Autodesk Fusion 360 part; units mm, degrees
note: some values were not read from the file. Set by a fixed rule: which sketch regions a step uses.
(part 2 of 2)
sketch "Sketch6" plane through (0, 2, 0) normal (0, 1, 0) x (-1, 0, 0) in component "Case"
  arc A0 (-13.01, 94.472) -> (-15.51, 96.972) centre (-15.51, 94.472) ccw
  line L0 (-13.01, 94.472) -> (-13.01, 43.354)
  arc A1 (-13.01, 43.354) -> (-11.51, 41.854) centre (-11.51, 43.354) ccw
  line L1 (-11.51, 41.854) -> (2.524, 41.854)
  arc A2 (5.024, 39.354) -> (2.524, 41.854) centre (2.524, 39.354) ccw
  line L2 (5.024, 39.354) -> (5.024, -2.524)
  arc A3 (2.524, -5.024) -> (5.024, -2.524) centre (2.524, -2.524) ccw
  line L3 (2.524, -5.024) -> (-93.964, -5.024)
  arc A4 (-96.464, -2.524) -> (-93.964, -5.024) centre (-93.964, -2.524) ccw
  line L4 (-96.464, -2.524) -> (-96.464, 94.472)
  arc A5 (-93.964, 96.972) -> (-96.464, 94.472) centre (-93.964, 94.472) ccw
  line L5 (-93.964, 96.972) -> (-15.51, 96.972)
  line L6 (-10.51, 44.354) -> (-10.51, 94.472)
  arc A6 (-10.51, 94.472) -> (-15.51, 99.472) centre (-15.51, 94.472) ccw
  line L7 (-15.51, 99.472) -> (-93.964, 99.472)
  arc A7 (-93.964, 99.472) -> (-98.964, 94.472) centre (-93.964, 94.472) ccw
  line L8 (-98.964, 94.472) -> (-98.964, -2.524)
  arc A8 (-98.964, -2.524) -> (-93.964, -7.524) centre (-93.964, -2.524) ccw
  line L9 (-93.964, -7.524) -> (2.524, -7.524)
  arc A9 (2.524, -7.524) -> (7.524, -2.524) centre (2.524, -2.524) ccw
  line L10 (7.524, -2.524) -> (7.524, 39.354)
  arc A10 (7.524, 39.354) -> (2.524, 44.354) centre (2.524, 39.354) ccw
  line L11 (2.524, 44.354) -> (-10.51, 44.354)
  line L12 (-12.247, -4.524) -> (-12.247, -2.174)
  line L13 (-3.247, -2.174) -> (-3.247, -4.524)
  line L14 (-3.247, -4.524) -> (2.524, -4.524)
  arc A11 (2.524, -4.524) -> (4.524, -2.524) centre (2.524, -2.524) ccw
  line L15 (4.524, -2.524) -> (4.524, 39.354)
  arc A12 (4.524, 39.354) -> (2.524, 41.354) centre (2.524, 39.354) ccw
  line L16 (2.524, 41.354) -> (-11.51, 41.354)
  arc A13 (-13.51, 43.354) -> (-11.51, 41.354) centre (-11.51, 43.354) ccw
  line L17 (-13.51, 43.354) -> (-13.51, 94.472)
  arc A14 (-13.51, 94.472) -> (-15.51, 96.472) centre (-15.51, 94.472) ccw
  line L18 (-15.51, 96.472) -> (-93.964, 96.472)
  arc A15 (-93.964, 96.472) -> (-95.964, 94.472) centre (-93.964, 94.472) ccw
  line L19 (-95.964, 94.472) -> (-95.964, -2.524)
  arc A16 (-95.964, -2.524) -> (-93.964, -4.524) centre (-93.964, -2.524) ccw
  line L20 (-93.964, -4.524) -> (-12.247, -4.524)
  line L21 (-90.666, 67.049) -> (-90.666, 82.049)
  line L22 (-90.666, 82.049) -> (-76.466, 82.049)
  line L23 (-76.466, 82.049) -> (-76.466, 67.049)
  line L24 (-76.466, 67.049) -> (-90.666, 67.049)
  circle A17 centre (-20.066, 74.613) radius 1.5875
  circle A18 centre (-89.408, 55.499) radius 1.5875
  line L25 (-52.966, 38.874) -> (-52.966, 53.074)
  line L26 (-52.966, 53.074) -> (-37.966, 53.074)
  line L27 (-37.966, 53.074) -> (-37.966, 38.874)
  line L28 (-37.966, 38.874) -> (-52.966, 38.874)
  line L29 (-72.016, 19.824) -> (-72.016, 34.024)
  line L30 (-72.016, 34.024) -> (-57.016, 34.024)
  line L31 (-57.016, 34.024) -> (-57.016, 19.824)
  line L32 (-57.016, 19.824) -> (-72.016, 19.824)
  line L33 (-37.966, 0.774) -> (-52.966, 0.774)
  line L34 (-52.966, 0.774) -> (-52.966, 14.974)
  line L35 (-52.966, 14.974) -> (-37.966, 14.974)
  line L36 (-37.966, 14.974) -> (-37.966, 0.774)
  line L37 (-72.016, 0.774) -> (-72.016, 14.974)
  line L38 (-72.016, 14.974) -> (-57.016, 14.974)
  line L39 (-57.016, 14.974) -> (-57.016, 0.774)
  line L40 (-57.016, 0.774) -> (-72.016, 0.774)
  line L41 (-52.966, 34.024) -> (-37.966, 34.024)
  line L42 (-37.966, 34.024) -> (-37.966, 19.824)
  line L43 (-37.966, 19.824) -> (-52.966, 19.824)
  line L44 (-52.966, 19.824) -> (-52.966, 34.024)
  line L45 (-72.016, 38.874) -> (-72.016, 53.074)
  line L46 (-72.016, 53.074) -> (-57.016, 53.074)
  line L47 (-57.016, 53.074) -> (-57.016, 38.874)
  line L48 (-57.016, 38.874) -> (-72.016, 38.874)
  line L49 (-72.016, 57.924) -> (-72.016, 72.124)
  line L50 (-72.016, 72.124) -> (-57.016, 72.124)
  line L51 (-57.016, 72.124) -> (-57.016, 57.924)
  line L52 (-57.016, 57.924) -> (-72.016, 57.924)
  line L53 (-33.916, 76.974) -> (-33.916, 91.174)
  line L54 (-33.916, 91.174) -> (-18.916, 91.174)
  line L55 (-18.916, 91.174) -> (-18.916, 76.974)
  line L56 (-18.916, 76.974) -> (-33.916, 76.974)
  line L57 (-72.016, 76.974) -> (-72.016, 91.174)
  line L58 (-72.016, 91.174) -> (-57.016, 91.174)
  line L59 (-57.016, 91.174) -> (-57.016, 76.974)
  line L60 (-57.016, 76.974) -> (-72.016, 76.974)
  line L61 (-33.916, 57.924) -> (-33.916, 72.124)
  line L62 (-33.916, 72.124) -> (-18.916, 72.124)
  line L63 (-18.916, 72.124) -> (-18.916, 57.924)
  line L64 (-18.916, 57.924) -> (-33.916, 57.924)
  line L65 (-90.666, 28.949) -> (-90.666, 43.949)
  line L66 (-90.666, 43.949) -> (-76.466, 43.949)
  line L67 (-76.466, 43.949) -> (-76.466, 28.949)
  line L68 (-76.466, 28.949) -> (-90.666, 28.949)
  line L69 (-33.916, 38.874) -> (-33.916, 53.074)
  line L70 (-33.916, 53.074) -> (-18.916, 53.074)
  line L71 (-18.916, 53.074) -> (-18.916, 38.874)
  line L72 (-18.916, 38.874) -> (-33.916, 38.874)
  circle A19 centre (-89.408, 17.399) radius 1.5875
  circle A20 centre (-35.941, 9.906) radius 1.5875
  line L73 (-33.916, 0.774) -> (-33.916, 14.974)
  line L74 (-33.916, 14.974) -> (-18.916, 14.974)
  line L75 (-18.916, 14.974) -> (-18.916, 0.774)
  line L76 (-18.916, 0.774) -> (-33.916, 0.774)
  line L77 (-91.066, 0.774) -> (-91.066, 14.974)
  line L78 (-91.066, 14.974) -> (-76.066, 14.974)
  line L79 (-76.066, 14.974) -> (-76.066, 0.774)
  line L80 (-76.066, 0.774) -> (-91.066, 0.774)
  line L81 (-33.916, 19.824) -> (-33.916, 34.024)
  line L82 (-33.916, 34.024) -> (-18.916, 34.024)
  line L83 (-18.916, 34.024) -> (-18.916, 19.824)
  line L84 (-18.916, 19.824) -> (-33.916, 19.824)
  circle A21 centre (-54.991, 55.499) radius 1.5875
  line L85 (-52.966, 57.924) -> (-52.966, 72.124)
  line L86 (-52.966, 72.124) -> (-37.966, 72.124)
  line L87 (-37.966, 72.124) -> (-37.966, 57.924)
  line L88 (-37.966, 57.924) -> (-52.966, 57.924)
  line L89 (-52.966, 76.974) -> (-52.966, 91.174)
  line L90 (-52.966, 91.174) -> (-37.966, 91.174)
  line L91 (-37.966, 91.174) -> (-37.966, 76.974)
  line L92 (-37.966, 76.974) -> (-52.966, 76.974)
  line L93 (-3.247, -2.174) -> (-12.247, -2.174)
  line L94 (-12.247, -2.174) -> (-12.247, -7.524) construction
  line L95 (-12.247, -7.524) -> (-3.247, -7.524)
  line L96 (-3.247, -7.524) -> (-3.247, -2.174) construction
  line L97 (-12.247, -2.174) -> (-17.414, -2.174)
  line L98 (-17.414, -2.174) -> (-17.414, 38.354)
  line L99 (-17.414, 38.354) -> (2.024, 38.354)
  line L100 (2.024, 38.354) -> (2.024, -2.174)
  line L101 (2.024, -2.174) -> (-3.247, -2.174)
  line L102 (-3.247, -7.524) -> (-12.247, -2.174) construction
  line L103 (-13.747, -2.174) -> (-1.747, -2.174)
  line L104 (-1.747, -2.174) -> (-1.747, -7.524)
  line L105 (-1.747, -7.524) -> (-13.747, -7.524)
  line L106 (-13.747, -7.524) -> (-13.747, -2.174)
  line L107 (-13.747, -2.174) -> (-1.747, -7.524) construction
  line L108 (-1.747, -2.174) -> (-13.747, -7.524) construction
  point P0 (-7.747, -4.849)
  dimension "d84" = 12
  dimension "d85" = 5.35
  constraint horizontal L93
  constraint vertical L94
  constraint horizontal L95
  constraint vertical L96
  constraint coincident L9 L94.end
  constraint coincident L13.start L93.start
  constraint coincident L12.end L93.end
  constraint perpendicular L103 L104
  constraint parallel L103 L105
  constraint parallel L104 L106
  constraint horizontal L103
  constraint coincident L107 P0
  constraint coincident L108 P0
  constraint midpoint L102 P0
  measures "d84" distance of L104.end L105.end
  measures "d85" distance of L103.end L104.end
extrude "Extrude6" cut sketch "Sketch6" against normal blind 8 contours L3 L12 L13 L14 L20 L93 L103 L104 L106 | L3 L9 L95 L104 L105 L106 | L12 L20 L97 L103 L106 | L13 L14 L101 L103 L104 bodies 2 in component "Case"
fillet "Fillet2" radius 2 13 edges at (-0.3885, 2, -7.524) (53.8555, 2, -7.524) (97.4995, 2, -6.0595) (98.964, 2, 45.974) (97.4995, 2, 98.0075) (54.737, 2, 99.472) (11.9745, 2, 98.0075) (10.51, 2, 69.413) (-0.3885, 2, -7.524) (-6.0595, 2, -6.0595) (-7.524, 2, 18.415) (-6.0595, 2, 42.8895) (3.993, 2, 44.354) on bodies 2 in component "Case"
sketch "Sketch1 (2)" plane through (0, -10, 0) normal (0, 1, 0) x (-1, 0, 0)
  circle A0 centre (-35.941, 9.906) radius 3.2553
  circle A1 centre (-54.991, 55.499) radius 3.2528
  line L0 (-15.51, 71.3577) -> (-20.066, 71.3577)
  arc A2 (-20.066, 77.8683) -> (-20.066, 71.3577) centre (-20.066, 74.613) ccw
  line L1 (-20.066, 77.8683) -> (-15.51, 77.8683)
  line L2 (-15.51, 77.8683) -> (-15.51, 91.694)
  arc A3 (-15.51, 91.694) -> (-18.288, 94.472) centre (-18.288, 91.694) ccw
  line L3 (-18.288, 94.472) -> (-91.44, 94.472)
  arc A4 (-91.44, 94.472) -> (-93.964, 91.948) centre (-91.44, 91.948) ccw
  line L4 (-93.964, 91.948) -> (-93.964, 58.7369)
  line L5 (-93.964, 58.7369) -> (-89.408, 58.7369)
  arc A5 (-89.408, 52.2611) -> (-89.408, 58.7369) centre (-89.408, 55.499) ccw
  line L6 (-89.408, 52.2611) -> (-93.964, 52.2611)
  line L7 (-93.964, 52.2611) -> (-93.964, 20.6443)
  line L8 (-93.964, 20.6443) -> (-89.408, 20.6443)
  arc A6 (-89.408, 14.1537) -> (-89.408, 20.6443) centre (-89.408, 17.399) ccw
  line L9 (-89.408, 14.1537) -> (-93.964, 14.1537)
  line L10 (-93.964, 14.1537) -> (-93.964, 0.254)
  arc A7 (-93.964, 0.254) -> (-91.186, -2.524) centre (-91.186, 0.254) ccw
  line L11 (-91.186, -2.524) -> (0, -2.524)
  arc A8 (0, -2.524) -> (2.524, 0) centre (0, 0) ccw
  line L12 (2.524, 0) -> (2.524, 37.084)
  arc A9 (2.524, 37.084) -> (0.254, 39.354) centre (0.254, 37.084) ccw
  line L13 (0.254, 39.354) -> (-15.24, 39.354)
  arc A10 (-15.51, 39.624) -> (-15.24, 39.354) centre (-15.24, 39.624) ccw
  line L14 (-15.51, 39.624) -> (-15.51, 71.3577)
  line L15 (-15.51, 39.624) -> (-15.51, -2.524)
  line L16 (-15.51, -2.524) -> (-93.2247, 93.7327) construction
  line L17 (-56.8674, 82.6104) -> (-56.8674, 18.55) construction
  arc A11 (-56.8674, 18.55) -> (-51.8674, 18.55) centre (-54.3674, 18.55) ccw construction
  line L18 (-51.8674, 18.55) -> (-51.8674, 82.6104) construction
  arc A12 (-51.8674, 82.6104) -> (-56.8674, 82.6104) centre (-54.3674, 82.6104) ccw construction
  line L19 (-54.3674, 82.6104) -> (-54.3674, 18.55) construction
  line L20 (-70.3674, 18.55) -> (-70.3674, 82.6104)
  arc A13 (-75.3674, 18.55) -> (-70.3674, 18.55) centre (-72.8674, 18.55) ccw
  line L21 (-75.3674, 82.6104) -> (-75.3674, 18.55)
  arc A14 (-70.3674, 82.6104) -> (-75.3674, 82.6104) centre (-72.8674, 82.6104) ccw
  line L22 (-33.3674, 18.55) -> (-33.3674, 82.6104)
  arc A15 (-38.3674, 18.55) -> (-33.3674, 18.55) centre (-35.8674, 18.55) ccw
  line L23 (-38.3674, 82.6104) -> (-38.3674, 18.55)
  arc A16 (-33.3674, 82.6104) -> (-38.3674, 82.6104) centre (-35.8674, 82.6104) ccw
  point P0 (-54.3674, 45.6044)
  point P1 (-54.3674, 50.5802)
  dimension "d92" = 5
  dimension "d95" = 18.5
  dimension "d96" = 0
  constraint coincident A10.start L14.start
  constraint coincident L11 L15.end
  constraint tangent A10 L15
  constraint midpoint A4 L16.end
  constraint midpoint L16 P0
  constraint tangent L17 A11
  constraint tangent A11 L18
  constraint parallel L17 L18
  constraint tangent L18 A12
  constraint tangent L17 A12
  constraint parallel L15 L19
  constraint midpoint L19 P1
  measures "d92" diameter of A11
extrude "Extrude7" cut sketch "Sketch1 (2)" against normal through all contours L20 A13 L21 A14 | L22 A15 L23 A16 bodies 2 in component "Case"
component "Plate" placed x (1, 0, 0) y (0, 1, 0) z (0, 0, 1) at (0, 0, 0)
component "Case" placed x (1, 0, 0) y (0, 1, 0) z (0, 0, 1) at (0, 0, 0)
equation "pcb_gap = 1 mm" comment "Gap between PCB and case"
equation "shoulder_width = 2 mm" comment "Shoulder width"
equation "plate_fillet = 2 mm" comment "Plate fillet radius"
equation "d5 = plate_fillet"
equation "d6 = plate_fillet"
equation "d7 = plate_fillet"
equation "d8 = plate_fillet"
equation "plate_thickness = 1.5 mm" comment "Plate thickness"
equation "d10 = plate_thickness"
equation "min_hole_radius = 3.175 mm" comment "Minimum hole radius"
equation "d13 = min_hole_radius"
equation "d14 = min_hole_radius"
equation "d15 = min_hole_radius"
equation "d16 = min_hole_radius"
equation "d17 = min_hole_radius"
equation "cherry_w = 15 mm" comment "Cherry MX hole width"
equation "cherry_h = 14.2 mm" comment "Cherry MX hole height"
equation "d23 = cherry_w"
equation "d24 = cherry_h"
equation "d25 = cherry_w"
equation "d26 = cherry_h"
equation "d27 = cherry_w"
equation "d28 = cherry_h"
equation "d29 = cherry_w"
equation "d30 = cherry_h"
equation "d31 = cherry_w"
equation "d32 = cherry_h"
equation "d33 = cherry_w"
equation "d34 = cherry_h"
equation "d35 = cherry_w"
equation "d36 = cherry_h"
equation "d37 = cherry_h"
equation "d38 = cherry_w"
equation "d39 = cherry_w"
equation "d40 = cherry_h"
equation "d41 = cherry_w"
equation "d42 = cherry_h"
equation "d43 = cherry_w"
equation "d44 = cherry_h"
equation "d45 = cherry_w"
equation "d46 = cherry_h"
equation "d47 = cherry_w"
equation "d48 = cherry_h"
equation "d49 = cherry_w"
equation "d50 = cherry_h"
equation "d51 = cherry_h"
equation "d52 = cherry_w"
equation "d53 = cherry_w"
equation "d54 = cherry_h"
equation "d55 = cherry_w"
equation "d56 = cherry_h"
equation "d57 = cherry_w"
equation "d58 = cherry_h"
equation "d66 = pcb_gap"
equation "d71 = min_hole_radius"
equation "d72 = min_hole_radius"
equation "d73 = min_hole_radius"
equation "d74 = min_hole_radius"
equation "d75 = min_hole_radius"
named bodies: "Plate", "Case"
